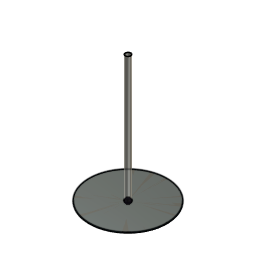
2022_12_26_Holder Sculture Jose v1 (Autodesk Fusion 360 design; units mm, degrees)
Autodesk Fusion 360 part; units mm, degrees
sketch "Sketch1" plane through (0, 0, 0) normal (0, 0, 1) x (1, 0, 0)
  circle A0 centre (0, 0) radius 55
  circle A1 centre (0, 0) radius 4
  circle A2 centre (0, 0) radius 3.15
  dimension "d1" = 110
  dimension "d2" = 8
  dimension "d3" = 6.3
  constraint coincident A0.centre A1.centre
  measures "d1" diameter of A0
  measures "d2" diameter of A1
  measures "d3" diameter of A2
extrude "Extrude1" add sketch "Sketch1" against normal blind 1 contours A0
extrude "Extrude2" add sketch "Sketch1" against normal blind 1 contours A1
extrude "Extrude3" add sketch "Sketch1" along normal blind 180 contours A1
equation "d3 = 8 mm - 1.7 mm"
